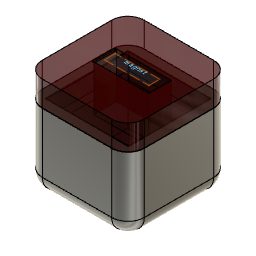
box v16 (Autodesk Fusion 360 design; units mm, degrees)
Autodesk Fusion 360 part; units mm, degrees
note: some values were not read from the file. Chosen so that the rebuilt part matches the saved one: which bodies a step acts on; which face or edge a step refers to.
sketch "Sketch1" plane through (0, 0, 0) normal (0, 0, 1) x (1, 0, 0)
  line L0 (0, 0) -> (75, 0)
  line L1 (75, 0) -> (75, 75)
  line L2 (75, 75) -> (0, 75)
  line L3 (0, 75) -> (0, 0)
  dimension "d1" = 75
  dimension "d2" = 75
  constraint horizontal L0
  constraint vertical L1
  constraint horizontal L2
  constraint vertical L3
  constraint coincident L0.start L3.end
  measures "d1" distance of L0.start L0.end
  measures "d2" distance of L0.start L2.end
extrude "Extrude1" add sketch "Sketch1" along normal blind 75 makes body 1
sketch "Sketch2" plane through (0, 0, 0) normal (0, -1, 0) x (1, 0, 0)
  line L0 (0, 0) -> (75, 0)
  line L1 (75, 0) -> (75, 75)
  line L2 (75, 75) -> (0, 75)
  line L3 (0, 75) -> (0, 0)
  line L4 (0, 56.3144) -> (75, 56.3144)
  constraint coincident L3 L4.start
  constraint perpendicular L3 L4
  constraint coincident L1 L4.end
split "Split1" by curves path "Sketch2" along L4 bodies 1 makes body 2 at (25, 50, 0)
shell "Shell1" thickness 7 removed faces 1 at (25, 50, 56.3144) on bodies 2
sketch "Sketch3" plane through (0, 0, 75) normal (0, 0, 1) x (-1, 0, 0)
  line L0 (0, -75) -> (0, 0)
  line L1 (0, 0) -> (-75, 0)
  line L2 (-75, 0) -> (-75, -75)
  line L3 (-75, -75) -> (0, -75)
  line L4 (-7.2828, -68.2159) -> (-68.4587, -68.2159)
  line L5 (-68.4587, -68.2159) -> (-68.4587, -7.7684)
  line L6 (-68.4587, -7.7684) -> (-7.2828, -7.7684)
  line L7 (-7.2828, -7.7684) -> (-7.2828, -68.2159)
  constraint horizontal L4
  constraint vertical L5
  constraint horizontal L6
  constraint vertical L7
sketch "Sketch4" plane through (0, 0, 56.3144) normal (0, 0, -1) x (1, 0, 0)
  line L0 (0, -75) -> (75, -75)
  line L1 (75, -75) -> (75, 0)
  line L2 (75, 0) -> (0, 0)
  line L3 (0, 0) -> (0, -75)
  line L4 (7.5507, -7.811) -> (68.2164, -7.811)
  line L5 (68.2164, -7.811) -> (68.2164, -67.956)
  line L6 (68.2164, -67.956) -> (7.5507, -67.956)
  line L7 (7.5507, -67.956) -> (7.5507, -7.811)
  constraint horizontal L4
  constraint vertical L5
  constraint horizontal L6
  constraint vertical L7
extrude "Extrude2" add sketch "Sketch4" along normal blind 15 contours L4 L5 L6 L7 bodies 1
fillet "Fillet1" radius 12 4 edges at (75, 0, 28.1572) (0, 0, 28.1572) (0, 37.5, 0) (75, 75, 28.1572) on bodies 2
fillet "Fillet2" radius 12 4 edges at (0, 75, 65.6572) (75, 75, 65.6572) (75, 0, 65.6572) (0, 0, 65.6572) on bodies 1
fillet "Fillet3" radius 12 8 edges at (3.5147, 3.5147, 3.5147) (37.5, 0, 0) (71.4853, 3.5147, 0) (75, 37.5, 0) (71.4853, 71.4853, 0) (37.5, 75, 0) (3.5147, 75, 3.5147) (0, 75, 34.1572) on bodies 2
sketch "Sketch5" plane through (0, 0, 75) normal (0, 0, 1) x (-1, 0, 0)
  arc A0 (0, -12) -> (-12, 0) centre (-12, -12) ccw
  line L0 (-12, 0) -> (-63, 0)
  arc A1 (-63, 0) -> (-75, -12) centre (-63, -12) ccw
  line L1 (-75, -12) -> (-75, -63)
  arc A2 (-75, -63) -> (-63, -75) centre (-63, -63) ccw
  line L2 (-63, -75) -> (-12, -75)
  arc A3 (-12, -75) -> (0, -63) centre (-12, -63) ccw
  line L3 (0, -63) -> (0, -12)
  line L4 (-18.8991, -46.2702) -> (-60, -46.2702)
  line L5 (-60, -46.2702) -> (-60, -30)
  line L6 (-60, -30) -> (-18.8991, -30)
  line L7 (-18.8991, -30) -> (-18.8991, -46.2702)
  constraint horizontal L4
  constraint vertical L5
  constraint horizontal L6
  constraint vertical L7
extrude "Extrude3" cut sketch "Sketch5" against normal blind 1 contours L4 L5 L6 L7 bodies 1
sketch "Sketch6" plane through (0, 0, 74) normal (0, 0, 1) x (-1, 0, 0)
  line L0 (-18.8991, -30) -> (-60, -30)
  line L1 (-60, -30) -> (-60, -46.2702)
  line L2 (-60, -46.2702) -> (-18.8991, -46.2702)
  line L3 (-18.8991, -46.2702) -> (-18.8991, -30)
  line L4 (-22.8093, -42.7945) -> (-55.6112, -42.7945)
  line L5 (-55.6112, -42.7945) -> (-55.6112, -34.757)
  line L6 (-55.6112, -34.757) -> (-22.8093, -34.757)
  line L7 (-22.8093, -34.757) -> (-22.8093, -42.7945)
  constraint horizontal L4
  constraint vertical L5
  constraint horizontal L6
  constraint vertical L7
extrude "Extrude4" add sketch "Sketch6" along normal blind 1 contours L4 L5 L6 L7 bodies 1
sketch "Sketch7" plane through (0, 0, 75) normal (0, 0, 1) x (-1, 0, 0)
  line L0 (-22.8093, -34.757) -> (-55.6112, -34.757)
  line L1 (-55.6112, -34.757) -> (-55.6112, -42.7945)
  line L2 (-55.6112, -42.7945) -> (-22.8093, -42.7945)
  line L3 (-22.8093, -42.7945) -> (-22.8093, -34.757)
  line L4 (-22.8093, -34.757) -> (-55.6112, -34.757) construction
  line L5 (-55.6112, -34.757) -> (-55.6112, -42.7945) construction
  line L6 (-55.6112, -42.7945) -> (-22.8093, -42.7945) construction
  line L7 (-22.8093, -42.7945) -> (-22.8093, -34.757) construction
  dimension "d18" = 3
  constraint coincident L0.end
  constraint coincident L2.end
chamfer "Chamfer1" distance 3 angle 45 4 edges at (68.2164, 37.8835, 41.3144) (37.8835, 7.811, 41.3144) (37.8835, 67.956, 41.3144) (7.5507, 37.8835, 41.3144) on bodies 1
sketch "Sketch8" plane through (0, 0, 41.3144) normal (0, 0, -1) x (1, 0, 0)
  line L0 (10.5507, -10.811) -> (10.5507, -64.956)
  line L1 (10.5507, -64.956) -> (65.2164, -64.956)
  line L2 (65.2164, -64.956) -> (65.2164, -10.811)
  line L3 (65.2164, -10.811) -> (10.5507, -10.811)
  line L4 (20, -30) -> (60.3555, -30)
  line L5 (60.3555, -30) -> (60.3555, -46.5696)
  line L6 (60.3555, -46.5696) -> (20, -46.5696)
  line L7 (20, -46.5696) -> (20, -30)
  constraint horizontal L4
  constraint vertical L5
  constraint horizontal L6
  constraint vertical L7
extrude "Extrude5" cut sketch "Sketch8" against normal blind 35 contours L4 L5 L6 L7 bodies 1
move_body "Move1" bodies 1 to x (1, 0, 0) y (0, 1, 0) z (0, 0, 1) at (0, 0, 25)
move_body "Move2" bodies 1 to x (1, 0, 0) y (0, 1, 0) z (0, 0, 1) at (-0.0477, 0, -25.3248)
equation "clearancefit = 0.5 mm"
equation "Transitionfit = 0.4 mm"
equation "Interferencefit = 0.3 mm"
named bodies: "lid"
